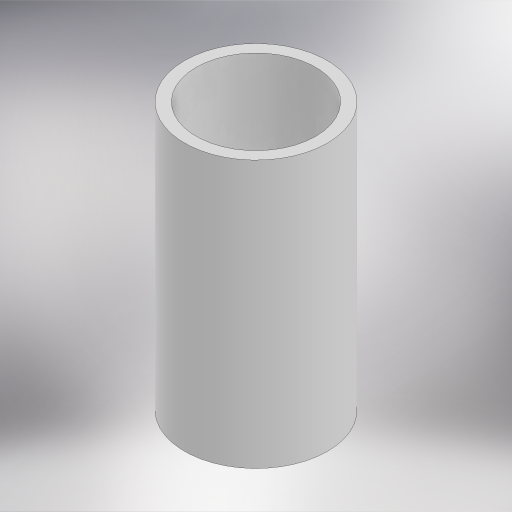
# Autodesk Inventor part: Tubo 12 40
Saved by Autodesk Inventor 2023 (Build 270158000, 158)
## iProperties
Created: 2023-02-27
Part Number: Tubo 12 40
Material: Genérico
Document SubType Name: Modeling
Designer: Braya
Density: 1 g/cm^3
Appearance: Valor por defecto
Author: Braya
Autodesk Inventor part; units mm, degrees
ref_plane "YZ Plane" through (0, 0, 0) normal (1, 0, 0) x (0, 1, 0)
ref_plane "XZ Plane" through (0, 0, 0) normal (0, 1, 0) x (-1, 0, 0)
ref_plane "XY Plane" through (0, 0, 0) normal (0, 0, 1) x (1, 0, 0)
sketch "Boceto2" plane through (0, 0, 0) normal (0, 1, 0) x (-1, 0, 0)
  circle A0 centre (0, 0) radius 8.96
  circle A1 centre (0, 0) radius 10.7
  dimension "d0" = 17.92
  dimension "d1" = 21.4
  constraints: 2 centre point, 2 coincident
  measures "d0" diameter of A0
  measures "d1" diameter of A1
extrude "Extrusión1" add sketch "Boceto2" along normal blind 40
